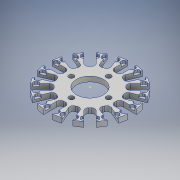
# Autodesk Inventor part: plate1_m6collet
Saved by Autodesk Inventor 2018 (Build 220112000, 112)
## iProperties
Created: 2017-08-17
Part Number: plate1_m6collet
Material: Aluminum 6061
Document SubType Name: Modeling
Designer: steve
Density: 2.7 g/cm^3
Appearance: Aluminum - Flat
Mass: 8.83202 g
Surface Area: 37.957 cm^2
Volume: 3.27112 cm^3
Author: steve
Autodesk Inventor part; units mm, degrees
ref_plane "YZ Plane" through (0, 0, 0) normal (1, 0, 0) x (0, 1, 0)
ref_plane "XZ Plane" through (0, 0, 0) normal (0, 1, 0) x (-1, 0, 0)
ref_plane "XY Plane" through (0, 0, 0) normal (0, 0, 1) x (1, 0, 0)
sketch "Sketch1" plane through (0, 0, 0) normal (0, 0, 1) x (1, 0, 0)
  circle A0 centre (0, 0) radius 25
  dimension "wheel_border" = 50
  constraints: 1 centre point, 1 coincident
  measures "wheel_border" diameter of A0
extrude "Extrusion1" add sketch "Sketch1" along normal blind 3
sketch "Sketch4" plane through (0, 0, 3) normal (0, 0, 1) x (1, 0, 0)
  line L0 (-35, 0) -> (35, 0) construction
  line L1 (0, -35) -> (0, 35) construction
  line L2 (-11.282, 25) -> (10.768, 25) construction
  line L3 (-11.9075, 22.5) -> (11.2763, 22.5) construction
  circle A0 centre (0, 0) radius 25 construction
  line L4 (4.075, 20.9625) -> (-4.075, 20.9625) construction
  line L5 (-4.075, 20.9625) -> (-4.075, 24.0375) construction
  line L6 (-4.075, 24.0375) -> (4.075, 24.0375) construction
  line L7 (4.075, 24.0375) -> (4.075, 20.9625) construction
  line L8 (4.075, 20.9625) -> (-4.075, 24.0375) construction
  line L9 (-4.075, 20.9625) -> (4.075, 24.0375) construction
  line L10 (4.075, 20.9625) -> (-4.075, 20.9625)
  line L11 (-4.075, 20.9625) -> (-4.075, 24.0375)
  line L12 (-4.075, 24.0375) -> (4.075, 24.0375)
  line L13 (4.075, 24.0375) -> (4.075, 20.9625)
  line L14 (4.075, 20.9625) -> (-4.075, 24.0375) construction
  line L15 (-4.075, 20.9625) -> (4.075, 24.0375) construction
  point P0 (0, 22.5)
  dimension "d23" = 2.5
  dimension "d24" = 3.075
  dimension "d25" = 8.15
  constraints: 28 end point, 4 horizontal, 4 midpoint, 4 parallel, 2 perpendicular, 2 point on line, 1 tangent
  measures "d23" distance between parallel lines of L3 L2
  measures "d24" distance of L6.end L4.start
  measures "d25" distance of L4.start L4.end
extrude "Extrusion4" cut sketch "Sketch4" against normal blind 1.5
sketch "Sketch5" plane through (0, 0, 3) normal (0, 0, 1) x (1, 0, 0)
  line L0 (-4.075, 20.9625) -> (-4.075, 24.0375) construction
  line L1 (4.075, 20.9625) -> (-4.075, 20.9625) construction
  line L2 (4.075, 24.0375) -> (4.075, 20.9625) construction
  line L3 (-4.075, 24.0375) -> (4.075, 24.0375) construction
  line L4 (-35, 0) -> (35, 0) construction
  line L5 (0, -35) -> (0, 35) construction
  line L6 (-4.075, 22.5) -> (4.075, 22.5) construction
  line L7 (4.075, 24.0375) -> (4.075, 20.9625) construction
  line L8 (2.575, 15) -> (-2.575, 15)
  line L9 (-2.575, 15) -> (-2.575, 30)
  line L10 (-2.575, 30) -> (2.575, 30)
  line L11 (2.575, 30) -> (2.575, 15)
  line L12 (2.575, 15) -> (-2.575, 30) construction
  line L13 (-2.575, 15) -> (2.575, 30) construction
  point P0 (0, 0)
  point P1 (0, 22.5)
  dimension "d28" = 15
  dimension "d29" = 5.15
  constraints: 14 end point, 5 midpoint, 2 parallel, 1 horizontal, 1 perpendicular
  measures "d28" distance of L10.end L8.start
  measures "d29" distance of L8.start L8.end
extrude "Extrusion5" cut sketch "Sketch5" against normal through all
fillet "Fillet2" radius 2 2 edges at (-2.575, 15, 1.5) (2.575, 15, 1.5)
fillet "Fillet3" radius 1 4 edges at (-4.075, 24.0375, 2.25) (-4.075, 20.9625, 2.25) (4.075, 24.0375, 2.25) (4.075, 20.9625, 2.25)
pattern_circular "Circular Pattern1" count 16 over 360 about axis through (0, 0, 0) along (0, 0, 1) of "Extrusion4", "Extrusion5", "Fillet2", "Fillet3"
sketch "Sketch6" plane through (0, 0, 0) normal (0, 0, -1) x (-1, 0, 0)
  circle A0 centre (0, 0) radius 8
  dimension "d37" = 16
  constraints: 1 centre point, 1 coincident
  measures "d37" diameter of A0
extrude "Extrusion6" cut sketch "Sketch6" against normal through all
sketch "Sketch7" plane through (0, 0, 0) normal (0, 0, -1) x (-1, 0, 0)
  circle A0 centre (0, 0) radius 11 construction
  point P0 (11, 0)
  point P1 (0, -11)
  point P2 (-11, 0)
  point P3 (0, 11)
  dimension "d40" = 22
  constraints: 4 point on circle, 1 centre point, 1 coincident
  measures "d40" diameter of A0
hole "Hole1" at (-11, 0, 0) at (0, -11, 0) at (11, 0, 0) at (0, 11, 0) direction (0, 0, 1) diameter 3 end through all
sketch "Sketch9" plane through (0, 0, 3) normal (0, 0, 1) x (1, 0, 0)
  point P0 (0, 0)
equation "\"d23\" = axis_to_border"
equation "\"d24\" = axis_w + 0.5 * fit_tol"
equation "\"d29\" = 2 * washer_w + bearing_w + fit_tol"
equation "\"fit_tol\" = 0.15"
equation "\"axis_w\" = 3"
equation "\"bearing_w\" = 4"
equation "\"washer_w\" = 0.5"
equation "\"bearing_l\" = 12"
equation "\"axis_to_border\" = 2.5"
body "Solid1"
